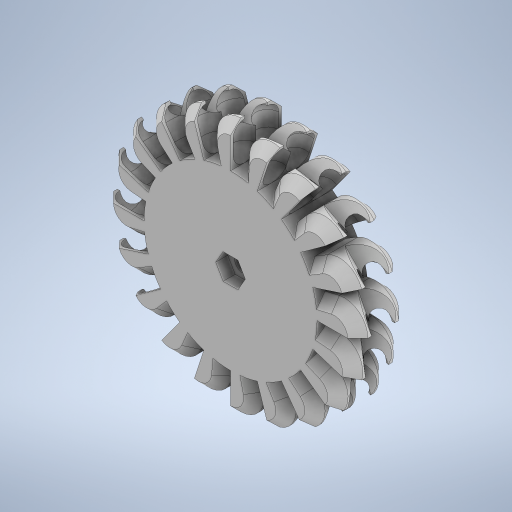
# Autodesk Inventor part: PeltonTurbine
Saved by Autodesk Inventor 2024.3 (Build 283343000, 343)
## iProperties
Created: 2024-12-10
Part Number: PeltonTurbine
Material: Generisch
Document SubType Name: Modeling
Designer: Maximilian Hock
Density: 1 g/cm^3
Appearance: Vorgabe
Author: Maximilian Hock
## iProperties of the stored document PeltonTurbine_3D-Druck.ipt
Created: 2025-01-13
Part Number: PeltonTurbine_3D-Druck
Material: Generisch
Document SubType Name: Modeling
Designer: Maximilian Hock
Density: 1 g/cm^3
Appearance: Vorgabe
Author: Maximilian Hock
Autodesk Inventor part; units mm, degrees
ref_plane "YZ Plane" through (0, 0, 0) normal (1, 0, 0) x (0, 1, 0)
sketch "Skizze5" plane through (0, 0, 0) normal (0, 1, 0) x (-1, 0, 0)
  line L0 (0, 0) -> (50, 0)
  line L1 (50, 0) -> (50, -11.5434) construction
  line L2 (50, -11.5434) -> (0, 0)
  arc A0 (38.7524, -8.9467) -> (50, 0) centre (40.818, 0) ccw
  line L3 (50, 0) -> (38.7524, -8.9467) construction
  arc A1 (38.7524, -8.9467) -> (39.7718, 0) centre (0, 0) ccw
  arc A2 (27.5066, -19.9847) -> (33.1286, -7.6483) centre (0, 0) ccw
  line L4 (0, 0) -> (27.5066, -19.9847)
  arc A3 (33.1286, -7.6483) -> (34, 0) centre (0, 0) ccw
  dimension "d22" = 50
  dimension "d23" = 13
  dimension "d61" = 16
  dimension "d65" = 36
  constraints: 10 end point, 9 point on circle, 4 centre point, 4 point on line, 3 coincident, 2 tangent, 1 horizontal, 1 perpendicular
  measures "d22" distance of L0.start L0.end
  measures "d23" angle of L0 L2
  measures "d61" distance of A3.end L0.end
  measures "d65" angle of L4 L0
extrude "Extrusion2" add sketch "Skizze5" along normal blind 10
sketch "Skizze6" plane through (-50, 0, 0) normal (0, 0, 1) x (1, 0, 0)
  line L0 (1, 4.5) -> (16, 4.5)
  arc A0 (1, 4.5) -> (5.5, 0) centre (5.5, 4.5) ccw
  arc A1 (11.5, 0) -> (16, 4.5) centre (11.5, 4.5) ccw
  line L1 (0, 0) -> (50, 0) projected
  line L2 (0, 0) -> (0, 10) projected
  arc A2 (5.5, 9) -> (1, 4.5) centre (5.5, 4.5) ccw construction
  line L3 (0, 10) -> (50, 10) construction
  dimension "d26" = 15
  dimension "d28" = 1
  dimension "d29" = 1
  constraints: 6 point on circle, 3 centre point, 3 tangent, 2 end point, 2 line through centre, 2 point on line, 1 coincident, 1 horizontal, 1 vertical alignment
  measures "d26" distance of L0.start L0.end
  measures "d28" distance from line of L2 L0.start
  measures "d29" distance from line of L3 A2.start
revolve "Umdrehung1" cut sketch "Skizze6" angle 360 about axis through (-49, 4.5, 0) along (1, 0, 0)
sketch "Skizze7" plane through (-38.5, 0, 0) normal (0, 0, 1) x (1, 0, 0)
  line L0 (-11.5, 10) -> (38.5, 10) projected
  line L1 (-11.5, 0) -> (-11.5, 10) projected
  line L2 (-11.5, 0) -> (-6, 0) projected
  arc A0 (-6, 9) -> (-6, 0) centre (-6, 4.5) ccw construction
  line L3 (-6, 9) -> (0, 9) projected
  arc A1 (0, 0) -> (0, 9) centre (0, 4.5) ccw projected
  line L4 (0, 0) -> (38.5, 0) projected
  line L5 (38.5, 0) -> (38.5, 10) projected
  line L6 (-11.5, 0) -> (-11.5, 5) projected
  line L7 (-10.5, 4.5) -> (-11.5, 4.5) construction
  arc A2 (-6, 10) -> (-11.5, 4.5) centre (-6, 4.5) ccw
  line L8 (4.5, 4.5) -> (4.5, 10)
  arc A3 (0, 0) -> (0, 9) centre (0, 4.5) ccw projected
  line L9 (4.5, 10) -> (-11.5, 10)
  line L10 (-11.5, 10) -> (-11.5, 19.2413)
  line L11 (-11.5, 19.2413) -> (4.5, 19.2413)
  line L12 (4.5, 19.2413) -> (4.5, 10)
  line L13 (-6, 0) -> (0, 0) projected
  line L14 (-6, 9) -> (-6, 0) projected
  line L15 (-6, 0) -> (-11.5, 4.5)
  constraints: 14 end point, 4 point on circle, 4 tangent, 3 point on line, 2 parallel, 2 perpendicular, 1 centre point, 1 horizontal, 1 vertical
extrude "Extrusion3" cut sketch "Skizze7" against normal through all draft 18 contours L15 L2 L1
ref_plane "Arbeitsebene3" through (-50, 0, 0) normal (1, 0, 0) x (0, 1, 0)
sketch "Skizze11" plane through (-50, 0, 0) normal (1, 0, 0) x (0, 1, 0)
  ellipse E0 centre (-3.0126, 0) end of major axis (-9.8397, 8.1964) minor radius 6.4666 (0, -9.1273) -> (4.5, 0) ccw projected
  line L0 (0, 0) -> (0, -9.1273) projected
  arc A0 (0, 0) -> (1.3485, -3.2122) centre (4.5, 0) ccw projected
  ellipse E1 centre (2.0619, -1.0236) end of major axis (3.2409, -3.8321) minor radius 1.8345 (1.3485, -3.2122) -> (3.6089, 0) ccw projected
  line L1 (4.5, 0) -> (3.6089, 0) projected
  ellipse E2 centre (2.0619, -1.0236) end of major axis (3.2409, -3.8321) minor radius 1.8345 (1.3485, -3.2122) -> (3.6089, 0) ccw projected
  line L2 (4.0845, -2.5537) -> (4.5, 0)
  line L3 (3.6089, 0) -> (9, 0) projected
  line L4 (4.5, 0) -> (3.6089, 0)
  line L5 (3.6089, 0) -> (4.0845, -2.5537)
  point P0 (0, 0)
  point P1 (4.5, 0)
  constraints: 6 end point, 1 coincident, 1 horizontal, 1 point on line, 5 other
extrude "Extrusion8" cut sketch "Skizze11" along normal up to surface contours L2 E1 L1 | E1 L5
sketch "Skizze10" plane through (-50, 10, 0) normal (0, 0, 1) x (1, 0, 0)
  arc A0 (11.5, -10) -> (11.5, -1) centre (11.5, -5.5) ccw projected
  line L0 (11.5, -10) -> (50, -10) projected
  line L1 (50, -10) -> (50, 0) projected
  line L2 (0, 0) -> (50, 0) projected
  arc A1 (5.5, -1) -> (1, -5.5) centre (5.5, -5.5) ccw projected
  line L3 (5.5, -1) -> (11.5, -1) projected
  line L4 (0, -5.5) -> (0, 0) projected
  ellipse E0 centre (3.5052, -7.9381) end of major axis (5.8627, -9.867) minor radius 0.9413 (5.5, -8.6515) -> (1.0891, -6.3911) ccw construction
  ellipse E1 centre (9.182, -13.0126) end of major axis (0.2126, -4.8493) minor radius 2.9184 (10.1833, -10) -> (0, -5.5) ccw construction
  line L5 (1.5103, -5.8763) -> (0.4599, -5.8763)
  line L6 (1.0891, -6.3911) -> (1.5103, -5.8763)
  line L7 (0, -5.5) -> (1, -5.5) projected
  point P0 (1.0974, -4.5688)
  point P1 (0, -4.5688)
  point P2 (11.2476, -8.8126)
  constraints: 4 end point, 2 horizontal, 1 point on circle, 1 point on line, 3 other
extrude "Extrusion7" [suppressed]
ref_plane "Arbeitsebene2" through (-44.5, 4.5, -5.5) normal (0, 1, 0) x (1, 0, 0)
chamfer "Fasen2" distance 4 angle 45 2 edges at (-35.9405, 10, -8.2975) (-46.5339, 10, -7.1859)
pattern_circular "Runde Anordnung2" count 20 over 360 about axis through (0, 0, 0) along (0, 1, 0)
mirror "Spiegeln2" about plane through (-25, 0, -4.591) normal (0, -1, 0)
sketch "Skizze8" plane through (-33.0224, -10, -23.9922) normal (0, -1, 0) x (0.5018404, 0, -0.8649602)
  line L0 (-10.0038, 40.6033) -> (-7.0921, 45.6466)
  line L1 (-7.0921, 45.6466) -> (-1.2686, 45.6466)
  line L2 (-1.2686, 45.6466) -> (1.6432, 40.6033)
  line L3 (1.6432, 40.6033) -> (-1.2686, 35.56)
  line L4 (-1.2686, 35.56) -> (-7.0921, 35.56)
  line L5 (-7.0921, 35.56) -> (-10.0038, 40.6033)
  circle A0 centre (-4.1803, 40.6033) radius 3.05
  dimension "d37" = 6.1
  dimension "d38" = 11.647
  constraints: 12 end point, 2 coincident, 1 centre point, 1 horizontal, 13 other
  measures "d37" diameter of A0
  measures "d38" distance of L2.end L0.start
extrude "Extrusion4" cut sketch "Skizze8" against normal blind 4.7 contours L0 L1 L2 L3 L4 L5 | A0
extrude "Extrusion5" cut sketch "Skizze8" against normal through all contours A0
equation "\"d22\" = 0.5 * TurbineDiameter"
equation "\"d37\" = AxleDiameter + Clearance"
equation "\"d38\" = HexnutOuterSize + Clearance"
equation "\"d39\" = HexnutHeight"
equation "\"TurbineDiameter\" = 100"
equation "\"AxleDiameter\" = 6"
equation "\"Clearance\" = 0.1"
equation "\"HexnutOuterSize\" = 11.547"
equation "\"HexnutHeight\" = 4.7"
